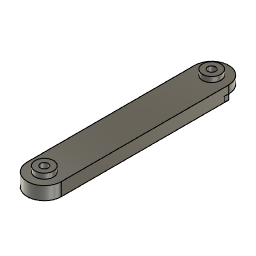
Barre Servo v4 (Autodesk Fusion 360 design; units mm, degrees)
Autodesk Fusion 360 part; units mm, degrees
note: some values were not read from the file. Set by a fixed rule: which sketch regions a step uses.
sketch "Esquisse1" plane through (0, 0, 0) normal (0, 0, 1) x (1, 0, 0)
  circle A0 centre (0, 0) radius 6.5
  circle A1 centre (0, 64) radius 6.5
  line L0 (0, 64) -> (0, 0)
  line L1 (0, 64) -> (-6.5, 64)
  line L2 (0, 64) -> (6.5, 64)
  line L3 (0, 0) -> (6.5, 0)
  line L4 (0, 0) -> (-6.5, 0)
  line L5 (-6.5, 64) -> (-6.5, 0)
  line L6 (6.5, 64) -> (6.5, 0)
  line L7 (0, 64) -> (0, 44.5)
  line L8 (-2.75, 47.25) -> (2.75, 47.25)
  circle A2 centre (0, 47.25) radius 2.75
  line L9 (-2.75, 47.25) -> (-6.3285, 62.5166)
  line L10 (2.75, 47.25) -> (6.3285, 62.5166)
  dimension "d1" = 13
  dimension "d2" = 13
  dimension "d3" = 64
  dimension "d4" = 19.5
  dimension "d5" = 5.5
  dimension "d6" = 2.75
  dimension "d7" = 2.75
  constraint coincident A0.centre L0.end
  constraint coincident A1.centre L0.start
  constraint vertical L0
  constraint coincident A1 L1.end
  constraint perpendicular L0 L1
  constraint coincident A1 L2.end
  constraint perpendicular L0 L2
  constraint coincident A0 L3.end
  constraint perpendicular L0 L3
  constraint coincident A0 L4.end
  constraint perpendicular L0 L4
  constraint coincident L0 L7.end
  constraint perpendicular L2 L7
  constraint perpendicular L5 L8
  constraint midpoint L8 A2.centre
  constraint coincident L8.end A2
  constraint coincident A1 L9.end
  constraint tangent A1 L9
  constraint coincident A1 L10.end
  constraint tangent A1 L10
  measures "d1" diameter of A0
  measures "d2" diameter of A1
  measures "d3" distance of A1.centre A0.centre
  measures "d4" distance of A1.centre L7.end
  measures "d5" distance of L8.start L8.end
  measures "d6" distance of L7 L8.end
  measures "d7" distance of L7.end L8
extrude "Extrusion1" add sketch "Esquisse1" along normal blind 3
extrude "Extrusion2" add sketch "Esquisse1" against normal blind 2 contours A0 L3 L4 | A0 A1 L0 L5 A2 L9 | A0 L0 L4 | A0 L0 L3 | A0 A1 L0 L6 A2 L10
sketch "Esquisse2" plane through (0, 0, 3) normal (0, 0, 1) x (-1, 0, 0)
  line L0 (6.5, -64) -> (6.5, 0)
  arc A0 (6.5, 0) -> (-6.5, 0) centre (0, 0) ccw
  line L1 (-6.5, 0) -> (-6.5, -64)
  arc A1 (-6.5, -64) -> (6.5, -64) centre (0, -64) ccw
  circle A2 centre (0, 0) radius 1.5
  circle A3 centre (0, -64) radius 1.5
  dimension "d12" = 3
  dimension "d13" = 3
  constraint concentric A0 A2
  constraint concentric A1 A3
  measures "d12" diameter of A2
  measures "d13" diameter of A3
extrude "Extrusion3" cut sketch "Esquisse2" against normal blind 5 contours A2 | A3
sketch "Esquisse3" plane through (0, 0, 3) normal (0, 0, 1) x (-1, 0, 0)
  circle A0 centre (0, -64) radius 1.5
  circle A1 centre (0, 0) radius 1.5
  line L0 (6.5, -64) -> (6.5, 0)
  arc A2 (6.5, 0) -> (-6.5, 0) centre (0, 0) ccw
  line L1 (-6.5, 0) -> (-6.5, -64)
  arc A3 (-6.5, -64) -> (6.5, -64) centre (0, -64) ccw
  circle A4 centre (0, -64) radius 1.5
  circle A5 centre (0, -64) radius 3.5
  circle A6 centre (0, 0) radius 1.5
  circle A7 centre (0, 0) radius 3.5
  dimension "d16" = 7
  dimension "d17" = 3
  dimension "d18" = 3
  dimension "d19" = 7
  constraint concentric A0 A4
  constraint concentric A4 A5
  constraint concentric A1 A6
  constraint concentric A6 A7
  measures "d16" diameter of A5
  measures "d17" diameter of A4
  measures "d18" diameter of A6
  measures "d19" diameter of A7
extrude "Extrusion5" add sketch "Esquisse3" along normal blind 2 contours A5 | A7
